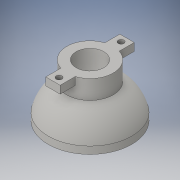
# Autodesk Inventor part: Sensing gripper
Saved by Autodesk Inventor 2016 (Build 200138000, 138)
## iProperties
Created: 2017-10-11
Part Number: Sensing gripper
Material: Generic
Document SubType Name: Modeling
Designer: ls769
Density: 1 g/cm^3
Appearance: Default
Author: ls769
Autodesk Inventor part; units mm, degrees
ref_plane "YZ Plane" through (0, 0, 0) normal (1, 0, 0) x (0, 1, 0)
ref_plane "XZ Plane" through (0, 0, 0) normal (0, 1, 0) x (-1, 0, 0)
ref_plane "XY Plane" through (0, 0, 0) normal (0, 0, 1) x (1, 0, 0)
sketch "Sketch1" plane through (0, 0, 0) normal (0, 0, 1) x (1, 0, 0)
  line L0 (22.5, 44) -> (22.5, 25.6111)
  line L1 (13.5, 44) -> (13.5, 29.9618)
  arc A0 (22.5, 18.6538) -> (13.5, 23.9242) centre (0, -9.4487) ccw
  arc A1 (34.7379, 0) -> (22.5, 18.6538) centre (0, -9.4487) ccw
  arc A2 (40.5729, 0) -> (22.5, 25.6111) centre (0, -9.4487) ccw
  line L2 (13.5, 29.9618) -> (13.5, 23.9242)
  line L3 (13.5, 44) -> (22.5, 44)
  line L4 (34.7379, 0) -> (40.5729, 0)
  line L5 (0, -20.1384) -> (0, 54.6897) projected
  point P0 (0, 0)
  constraints: 10 end point, 6 point on circle, 3 centre point, 1 coincident, 1 horizontal, 1 parallel
revolve "Revolution1" add sketch "Sketch1" angle 360 about axis through (0, -10, 0) along (0, 1, 0)
sketch "Sketch2" plane through (0, 44, 0) normal (0, 1, 0) x (1, 0, 0)
  line L0 (-7, -13.5) -> (-7, -36)
  line L1 (-7, -36) -> (7, -36)
  line L2 (7, -36) -> (7, -13.5)
  line L3 (7, -13.5) -> (7, -11.5434)
  circle A0 centre (0, 0) radius 13.5 projected
  line L4 (-7, -13.5) -> (-7, -11.5434)
  line L5 (-7, 13.5) -> (-7, 36)
  line L6 (-7, 36) -> (7, 36)
  line L7 (7, 36) -> (7, 13.5)
  line L8 (-7, 13.5) -> (-7, 11.5434)
  line L9 (7, 13.5) -> (7, 11.5434)
  dimension "d12" = 14
  dimension "d13" = 22.5
  dimension "d16" = 14
  dimension "d17" = 22.5
  constraints: 20 end point, 4 parallel, 4 point on circle, 2 vertical
  measures "d12" distance of L1.end L0.end
  measures "d13" distance of L0.end L0.start
  measures "d16" distance of L5.end L6.end
  measures "d17" distance of L5.start L5.end
extrude "Extrusion1" add sketch "Sketch2" against normal blind 7.5 contours L4 A0 L3 L2 L1 L0 | L8 L5 L6 L7 L9 A0
sketch "Sketch3" plane through (-7, 44, -36) normal (0, 1, 0) x (1, 0, 0)
  circle A0 centre (7, -66.0778) radius 2.8
  circle A1 centre (7.0706, -5.9222) radius 2.8
  line L0 (14, -14.6166) -> (14, 0) projected
  point P0 (7, -36)
  dimension "d20" = 5.6
  dimension "d21" = 5.6
  constraints: 2 centre point
  measures "d20" diameter of A0
  measures "d21" diameter of A1
extrude "Extrusion2" cut sketch "Sketch3" against normal blind 7.5
sketch "Sketch4" plane through (0, 0, 0) normal (0, -1, 0) x (1, 0, 0)
  circle A0 centre (0, 0) radius 40.5729
  constraints: 1 centre point, 1 coincident
extrude "Extrusion3" add sketch "Sketch4" along normal blind 7
sketch "Sketch5" plane through (0, -7, 0) normal (0, -1, 0) x (1, 0, 0)
  arc A0 (16.1775, -12.0133) -> (16.301, -12.0133) centre (16.2392, -12.0133) ccw
  arc A1 (16.301, -12.0133) -> (16.1775, -12.0133) centre (16.2392, -12.0133) ccw
  arc A2 (23.9531, -12.0133) -> (24.0765, -12.0133) centre (24.0148, -12.0133) ccw
  arc A3 (24.0765, -12.0133) -> (23.9531, -12.0133) centre (24.0148, -12.0133) ccw
  arc A4 (24.0148, -12.0133) -> (16.2392, -12.0133) centre (20.127, -12.0133) ccw
  arc A5 (16.2392, -12.0133) -> (24.0148, -12.0133) centre (20.127, -12.0133) ccw
  arc A6 (19.3718, -10.1309) -> (11.5963, -10.1309) centre (15.484, -10.1309) ccw
  arc A7 (11.5963, -10.1309) -> (19.3718, -10.1309) centre (15.484, -10.1309) ccw
  arc A8 (19.3101, -10.1309) -> (19.4335, -10.1309) centre (19.3718, -10.1309) ccw
  arc A9 (19.4335, -10.1309) -> (19.3101, -10.1309) centre (19.3718, -10.1309) ccw
  arc A10 (12.4208, 8.2206) -> (12.5442, 8.2206) centre (12.4825, 8.2206) ccw
  arc A11 (12.5442, 8.2206) -> (12.4208, 8.2206) centre (12.4825, 8.2206) ccw
  arc A12 (20.1963, 8.2206) -> (20.3198, 8.2206) centre (20.2581, 8.2206) ccw
  arc A13 (20.3198, 8.2206) -> (20.1963, 8.2206) centre (20.2581, 8.2206) ccw
  arc A14 (16.3725, 11.3003) -> (16.496, 11.3003) centre (16.4342, 11.3003) ccw
  arc A15 (16.496, 11.3003) -> (16.3725, 11.3003) centre (16.4342, 11.3003) ccw
  arc A16 (20.2581, 8.2206) -> (12.4825, 8.2206) centre (16.3703, 8.2206) ccw
  arc A17 (12.4825, 8.2206) -> (20.2581, 8.2206) centre (16.3703, 8.2206) ccw
  arc A18 (24.1481, 11.3003) -> (24.2715, 11.3003) centre (24.2098, 11.3003) ccw
  arc A19 (24.2715, 11.3003) -> (24.1481, 11.3003) centre (24.2098, 11.3003) ccw
  arc A20 (24.2098, 11.3003) -> (16.4342, 11.3003) centre (20.322, 11.3003) ccw
  arc A21 (16.4342, 11.3003) -> (24.2098, 11.3003) centre (20.322, 11.3003) ccw
  arc A22 (-16.4271, -11.6758) -> (-16.3037, -11.6758) centre (-16.3654, -11.6758) ccw
  arc A23 (-16.3037, -11.6758) -> (-16.4271, -11.6758) centre (-16.3654, -11.6758) ccw
  arc A24 (-12.4137, -8.5961) -> (-20.1892, -8.5961) centre (-16.3014, -8.5961) ccw
  arc A25 (-20.1892, -8.5961) -> (-12.4137, -8.5961) centre (-16.3014, -8.5961) ccw
  arc A26 (-20.2509, -8.5961) -> (-20.1275, -8.5961) centre (-20.1892, -8.5961) ccw
  arc A27 (-20.1275, -8.5961) -> (-20.2509, -8.5961) centre (-20.1892, -8.5961) ccw
  arc A28 (-12.4754, -8.5961) -> (-12.3519, -8.5961) centre (-12.4137, -8.5961) ccw
  arc A29 (-12.3519, -8.5961) -> (-12.4754, -8.5961) centre (-12.4137, -8.5961) ccw
  arc A30 (3.7067, -23.2293) -> (-4.0688, -23.2293) centre (-0.181, -23.2293) ccw
  arc A31 (-4.0688, -23.2293) -> (3.7067, -23.2293) centre (-0.181, -23.2293) ccw
  arc A32 (3.0359, -18.5391) -> (-4.7397, -18.5391) centre (-0.8519, -18.5391) ccw
  arc A33 (-4.7397, -18.5391) -> (3.0359, -18.5391) centre (-0.8519, -18.5391) ccw
  arc A34 (-24.2027, -11.6758) -> (-24.0792, -11.6758) centre (-24.1409, -11.6758) ccw
  arc A35 (-24.0792, -11.6758) -> (-24.2027, -11.6758) centre (-24.1409, -11.6758) ccw
  arc A36 (-16.3654, -11.6758) -> (-24.1409, -11.6758) centre (-20.2532, -11.6758) ccw
  arc A37 (-24.1409, -11.6758) -> (-16.3654, -11.6758) centre (-20.2532, -11.6758) ccw
  arc A38 (-19.365, 9.7553) -> (-19.2416, 9.7553) centre (-19.3033, 9.7553) ccw
  arc A39 (-19.2416, 9.7553) -> (-19.365, 9.7553) centre (-19.3033, 9.7553) ccw
  arc A40 (-11.5277, 9.7553) -> (-19.3033, 9.7553) centre (-15.4155, 9.7553) ccw
  arc A41 (-19.3033, 9.7553) -> (-11.5277, 9.7553) centre (-15.4155, 9.7553) ccw
  arc A42 (-11.5894, 9.7553) -> (-11.466, 9.7553) centre (-11.5277, 9.7553) ccw
  arc A43 (-11.466, 9.7553) -> (-11.5894, 9.7553) centre (-11.5277, 9.7553) ccw
  arc A44 (-24.008, 11.6378) -> (-23.8845, 11.6378) centre (-23.9462, 11.6378) ccw
  arc A45 (-23.8845, 11.6378) -> (-24.008, 11.6378) centre (-23.9462, 11.6378) ccw
  arc A46 (-16.1707, 11.6378) -> (-23.9462, 11.6378) centre (-20.0585, 11.6378) ccw
  arc A47 (-23.9462, 11.6378) -> (-16.1707, 11.6378) centre (-20.0585, 11.6378) ccw
  arc A48 (-16.2324, 11.6378) -> (-16.109, 11.6378) centre (-16.1707, 11.6378) ccw
  arc A49 (-16.109, 11.6378) -> (-16.2324, 11.6378) centre (-16.1707, 11.6378) ccw
  arc A50 (-3.7405, 23.3979) -> (-3.617, 23.3979) centre (-3.6788, 23.3979) ccw
  arc A51 (-3.617, 23.3979) -> (-3.7405, 23.3979) centre (-3.6788, 23.3979) ccw
  arc A52 (4.0351, 23.3979) -> (4.1585, 23.3979) centre (4.0968, 23.3979) ccw
  arc A53 (4.1585, 23.3979) -> (4.0351, 23.3979) centre (4.0968, 23.3979) ccw
  arc A54 (4.0968, 23.3979) -> (-3.6788, 23.3979) centre (0.209, 23.3979) ccw
  arc A55 (-3.6788, 23.3979) -> (4.0968, 23.3979) centre (0.209, 23.3979) ccw
  arc A56 (-3.0289, 18.1638) -> (-2.9055, 18.1638) centre (-2.9672, 18.1638) ccw
  arc A57 (-2.9055, 18.1638) -> (-3.0289, 18.1638) centre (-2.9672, 18.1638) ccw
  arc A58 (4.7467, 18.1638) -> (4.8701, 18.1638) centre (4.8084, 18.1638) ccw
  arc A59 (4.8701, 18.1638) -> (4.7467, 18.1638) centre (4.8084, 18.1638) ccw
  arc A60 (4.8084, 18.1638) -> (-2.9672, 18.1638) centre (0.9206, 18.1638) ccw
  arc A61 (-2.9672, 18.1638) -> (4.8084, 18.1638) centre (0.9206, 18.1638) ccw
  constraints: 124 point on circle, 62 centre point
extrude "Extrusion4" cut sketch "Sketch5" against normal blind 1 contours A0 A5 A7 A6 A4 A1 | A5 A4 A1 A0 | A0 A1 A4 A6 A9 A8 A7 A5 | A7 A8 A9 A6 A4 A3 A2 A5 | A2 A3 A4 A5 | A8 A9 A6 A7 | A17 A16 A11 A10 | A10 A11 A16 A20 A15 A14 A21 A17 | A21 A14 A15 A20 A16 A13 A12 A17 | A17 A12 A13 A16 A20 A19 A18 A21 | A12 A13 A16 A17 | A21 A20 A15 A14 | A18 A19 A20 A21 | A23 A36 A37 A22 | A22 A37 A25 A26 A27 A24 A36 A23 | A22 A23 A36 A24 A29 A28 A25 A37 | A37 A34 A35 A36 A24 A27 A26 A25 | A25 A24 A27 A26 | A28 A29 A24 A25 | A37 A36 A35 A34 | A31 A30 A33 | A33 A30 | A30 A33 A32 | A38 A41 A47 A44 A45 A46 A40 A39 | A41 A40 A39 A38 | A38 A39 A40 A46 A49 A48 A47 A41 | A47 A48 A49 A46 A40 A43 A42 A41 | A42 A43 A40 A41 | A47 A46 A45 A44 | A48 A49 A46 A47 | A55 A54 A51 A50 | A50 A51 A54 A53 A52 A55 A60 | A60 A55 | A55 A60 A59 A58 A61 A56 A57 | A54 A55 A52 A53 | A57 A56 A61 A60 | A60 A61 A58 A59 picked at (16.2777, -12.003) picked at (23.9764, -12.0235) picked at (19.3334, -10.1207) picked at (12.5209, 8.2104) picked at (20.2196, 8.2103) picked at (16.4727, 11.3106) picked at (24.1714, 11.2901) picked at (-16.4038, -11.6656) picked at (-20.1508, -8.6063) picked at (-12.4521, -8.5859) picked at (-24.1025, -11.686) picked at (-19.2649, 9.7655) picked at (-11.5661, 9.7451) picked at (-23.9078, 11.6276) picked at (-16.2091, 11.648) picked at (-3.6403, 23.4082) picked at (4.0584, 23.4081) picked at (-2.9288, 18.1536) picked at (4.77, 18.174)
sketch "Sketch6" plane through (0, -7, 0) normal (0, -1, 0) x (1, 0, 0)
  point P0 (0, 0)
sketch "Sketch7" plane through (0, -7, 0) normal (0, -1, 0) x (1, 0, 0)
  point P0 (0, 0)
sketch "Sketch8" plane through (0, -7, 0) normal (0, -1, 0) x (1, 0, 0)
  point P0 (0, 0)
body "Solid1"
